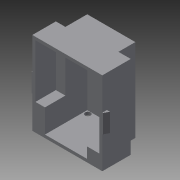
# Autodesk Inventor part: SkateBox
Saved by Autodesk Inventor 2013 (Build 170138000, 138)
## iProperties
Created: 2015-10-02
Part Number: SkateBox
Material: Generic
Document SubType Name: Modeling
Designer: A.Barredo
Density: 1 g/cm^3
Author: A.Barredo
Autodesk Inventor part; units mm, degrees
ref_plane "YZ Plane" through (0, 0, 0) normal (1, 0, 0) x (0, 1, 0)
ref_plane "XZ Plane" through (0, 0, 0) normal (0, 1, 0) x (-1, 0, 0)
ref_plane "XY Plane" through (0, 0, 0) normal (0, 0, 1) x (1, 0, 0)
sketch "Sketch1" plane through (0, 0, 0) normal (0, 0, 1) x (1, 0, 0)
  line L0 (-9.6334, 0) -> (35.8666, 0)
  line L1 (35.8666, 0) -> (35.8666, 18.5)
  line L2 (35.8666, 18.5) -> (27.8666, 18.5)
  line L3 (27.8666, 18.5) -> (27.8666, 29.5)
  line L4 (27.8666, 29.5) -> (-3.4334, 29.5)
  line L5 (-3.4334, 29.5) -> (-3.4334, 15.3)
  line L6 (-3.4334, 15.3) -> (-9.6334, 15.3)
  line L7 (-9.6334, 0) -> (-9.6334, 15.3)
  point P0 (0, 0)
  dimension "d0" = 45.5
  dimension "d1" = 18.5
  dimension "d2" = 8
  dimension "d3" = 11
  dimension "d4" = 31.3
  dimension "d5" = 14.2
  dimension "d6" = 6.2
  constraints: 16 end point, 5 parallel, 1 horizontal, 1 perpendicular
  measures "d0" distance of L0.start L0.end
  measures "d1" distance of L0.end L1.end
  measures "d2" distance of L1.end L2.end
  measures "d3" distance of L2.end L3.end
  measures "d4" distance of L3.end L4.end
  measures "d5" distance of L4.end L5.end
  measures "d6" distance of L5.end L6.end
extrude "Extrusion1" add sketch "Sketch1" against normal blind 52
shell "Shell1" thickness 2 removed faces 1 at (7.5999, 5.1, 0)
sketch "Sketch2" plane through (-7.6334, 2, -50) normal (0, 0, 1) x (1, 0, 0)
  line L0 (41.5, 0) -> (0, 0) projected
  line L1 (0, 11.3) -> (6.2, 11.3)
  line L2 (6.2, 11.3) -> (6.2, 0)
  line L3 (6.2, 0) -> (0, 0)
  line L4 (0, 0) -> (0, 11.3)
  point P0 (7.6334, -2)
  constraints: 8 end point, 2 parallel, 1 horizontal, 1 perpendicular, 1 point on line
extrude "Extrusion2" add sketch "Sketch2" along normal blind 15.3
sketch "Sketch3" plane through (-1.4334, 2, -50) normal (0, 0, 1) x (1, 0, 0)
  line L0 (35.3, 0) -> (0, 0) projected
  line L1 (35.3, 14.5) -> (27.3, 14.5)
  line L2 (27.3, 14.5) -> (27.3, 0)
  line L3 (27.3, 0) -> (35.3, 0)
  line L4 (35.3, 0) -> (35.3, 14.5)
  point P0 (1.4334, -2)
  constraints: 8 end point, 2 parallel, 1 horizontal, 1 perpendicular, 1 point on line
extrude "Extrusion3" add sketch "Sketch3" along normal blind 7
sketch "Sketch4" plane through (0, 0, 0) normal (0, 0, 1) x (1, 0, 0)
  line L0 (-9.6334, 0) -> (35.8666, 0) projected
  line L1 (-7.6334, 2) -> (33.8666, 2)
  line L2 (33.8666, 2) -> (33.8666, 0)
  line L3 (33.8666, 0) -> (-7.6334, 0)
  line L4 (-7.6334, 0) -> (-7.6334, 2)
  point P0 (0, 0)
  constraints: 8 end point, 2 parallel, 1 horizontal, 1 perpendicular, 1 point on line
extrude "Extrusion4" cut sketch "Sketch4" against normal blind 151
sketch "Sketch5" plane through (-7.6334, 2, -52) normal (0, -1, 0) x (1, 0, 0)
  line L0 (41.5, 0) -> (0, 0) projected
  line L1 (41.5, 9) -> (41.5, 0) projected
  line L2 (41.5, 9) -> (33.5, 9) projected
  line L3 (33.5, 9) -> (33.5, 2) projected
  line L4 (33.5, 2) -> (6.2, 2) projected
  line L5 (6.2, 2) -> (6.2, 17.3) projected
  line L6 (6.2, 17.3) -> (0, 17.3) projected
  line L7 (0, 17.3) -> (0, 0) projected
  point P0 (7.6334, 52)
extrude "Extrusion5" add sketch "Sketch5" along normal blind 2
sketch "Sketch6" plane through (0, 0, 0) normal (0, 0, 1) x (1, 0, 0)
  line L0 (-3.4334, 29.5) -> (27.8666, 29.5)
  line L1 (27.8666, 29.5) -> (27.8666, 0)
  line L2 (27.8666, 0) -> (-3.4334, 0)
  line L3 (-3.4334, 0) -> (-3.4334, 29.5)
  line L4 (-9.6334, 15.3) -> (-3.4334, 15.3)
  line L5 (-3.4334, 15.3) -> (-3.4334, 0)
  line L6 (-3.4334, 0) -> (-9.6334, 0)
  line L7 (-9.6334, 0) -> (-9.6334, 15.3)
  line L8 (27.8666, 18.5) -> (35.8666, 18.5)
  line L9 (35.8666, 18.5) -> (35.8666, 0)
  line L10 (35.8666, 0) -> (27.8666, 0)
  line L11 (27.8666, 0) -> (27.8666, 18.5)
  point P0 (0, 0)
  constraints: 24 end point, 6 parallel, 3 horizontal, 3 perpendicular
extrude "Extrusion6" add sketch "Sketch6" along normal blind 2
sketch "Sketch7" plane through (-9.6334, 0, -52) normal (-1, 0, 0) x (0, 0, 1)
  line L0 (0, 0) -> (0, 15.3) projected
  line L1 (54, 0) -> (0, 0) projected
  line L2 (21, 0) -> (33, 0)
  line L3 (33, 0) -> (33, 4.0069)
  line L4 (33, 4.0069) -> (21, 4.0069)
  line L5 (21, 4.0069) -> (21, 0)
  point P0 (52, 0)
  dimension "d20" = 54
  dimension "d21" = 12
  dimension "d22" = 21
  constraints: 8 end point, 2 parallel, 1 horizontal, 1 perpendicular, 1 point on line
  measures "d20" distance of L1.start L0.start
  measures "d21" distance of L3.end L4.end
  measures "d22" distance between parallel lines of L5 L0
extrude "Extrusion7" add sketch "Sketch7" along normal blind 2
sketch "Sketch8" plane through (-9.6334, 0, -52) normal (0, -1, 0) x (1, 0, 0)
  line L0 (45.5, 0) -> (45.5, 54) projected
  line L1 (45.5, 33) -> (47.5, 33)
  line L2 (47.5, 33) -> (47.5, 21)
  line L3 (47.5, 21) -> (45.5, 21)
  line L4 (45.5, 21) -> (45.5, 33)
  point P0 (9.6334, 52)
  dimension "d25" = 2
  constraints: 8 end point, 2 parallel, 1 horizontal, 1 perpendicular, 1 point on line
  measures "d25" distance of L2.end L3.end
extrude "Extrusion8" add sketch "Sketch8" against normal blind 3
sketch "Sketch9" plane through (35.8666, 0, -19) normal (0, 0, 1) x (1, 0, 0)
  line L0 (2, 0) -> (0, 0) projected
  line L1 (2, 0) -> (2, 3) projected
  line L2 (0, 0) -> (0, 3) projected
  line L3 (0.454, 0) -> (2, 3)
  line L4 (2, 3) -> (2, 0)
  point P0 (-35.8666, 0)
  constraints: 4 end point, 1 parallel, 1 point on line
extrude "Extrusion9" cut sketch "Sketch9" against normal blind 19.25
sketch "Sketch10" plane through (-9.6334, 0, -19) normal (0, 0, 1) x (1, 0, 0)
  line L0 (-2, 0) -> (-2, 4.0069) projected
  line L1 (0, 0) -> (-2, 0) projected
  line L2 (0, 0) -> (-0.454, 0)
  line L3 (-0.454, 0) -> (-2, 4.0069)
  line L4 (-2, 0) -> (-0.454, 0)
  line L5 (-2, 0) -> (-2, 4.0069)
  point P0 (9.6334, 0)
  dimension "d30" = 0.454
  constraints: 8 end point, 2 perpendicular, 1 point on line
  measures "d30" distance of L1.start L2.end
extrude "Extrusion10" cut sketch "Sketch10" against normal blind 34.5
sketch "Sketch11" plane through (0, 0, -52) normal (0, 0, -1) x (-1, 0, 0)
  circle A0 centre (-0.9313, 25.5293) radius 1.7905
  point P0 (0, 0)
  constraints: 1 centre point
extrude "Extrusion11" cut sketch "Sketch11" against normal blind 27.25
body "Solid1"
